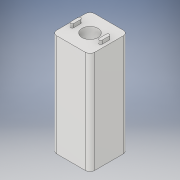
# Autodesk Inventor part: Camera Mount 30mm
Saved by Autodesk Inventor 2019 (Build 230136000, 136)
## iProperties
Created: 2020-02-21
Part Number: Camera Mount 30mm
Material: Generic
Document SubType Name: Modeling
Designer: close
Density: 1 g/cm^3
Appearance: Smooth - White
Author: close
Autodesk Inventor part; units mm, degrees
ref_plane "YZ Plane" through (0, 0, 0) normal (1, 0, 0) x (0, 1, 0)
ref_plane "XZ Plane" through (0, 0, 0) normal (0, 1, 0) x (-1, 0, 0)
ref_plane "XY Plane" through (0, 0, 0) normal (0, 0, 1) x (1, 0, 0)
sketch "Sketch1" plane through (0, 0, 0) normal (0, 1, 0) x (-1, 0, 0)
  line L0 (6, 8) -> (-6, 8)
  line L1 (-8, 6) -> (-8, -6)
  line L2 (-6, -8) -> (6, -8)
  line L3 (8, -6) -> (8, 6)
  arc A0 (8, 6) -> (6, 8) centre (6, 6) ccw
  arc A1 (-6, 8) -> (-8, 6) centre (-6, 6) ccw
  arc A2 (-8, -6) -> (-6, -8) centre (-6, -6) ccw
  arc A3 (6, -8) -> (8, -6) centre (6, -6) ccw
  point P0 (0, 0)
  point P1 (8, 8)
  point P2 (-8, 8)
  point P3 (8, -8)
  dimension "d0" = 16
  dimension "d1" = 16
  dimension "d2" = 8
  dimension "d3" = 8
  dimension "d4" = 2
  constraints: 8 end point, 8 point on circle, 8 tangent, 6 point on line, 4 centre point, 3 equal radius, 2 parallel, 1 horizontal, 1 perpendicular
  measures "d0" distance of point (8, -8) point (8, 8)
  measures "d1" distance of point (8, 8) point (-8, 8)
  measures "d2" distance from line of L0 point (0, 0)
  measures "d3" distance from line of point (0, 0) L3
  measures "d4" radius of A0
extrude "Extrusion1" add sketch "Sketch1" along normal blind 43
sketch "Sketch2" plane through (0, 0, 0) normal (0, -1, 0) x (1, 0, 0)
  line L0 (-6, 5.875) -> (-6, 3.125) construction
  line L1 (-7.375, 5.875) -> (-7.375, 3.125)
  line L2 (-4.625, 3.125) -> (-4.625, 5.875)
  arc A0 (-4.625, 5.875) -> (-7.375, 5.875) centre (-6, 5.875) ccw
  arc A1 (-7.375, 3.125) -> (-4.625, 3.125) centre (-6, 3.125) ccw
  line L3 (6, -3.125) -> (6, -5.875) construction
  line L4 (4.625, -3.125) -> (4.625, -5.875)
  line L5 (7.375, -5.875) -> (7.375, -3.125)
  arc A2 (7.375, -3.125) -> (4.625, -3.125) centre (6, -3.125) ccw
  arc A3 (4.625, -5.875) -> (7.375, -5.875) centre (6, -5.875) ccw
  point P0 (0, 0)
  point P1 (0, 0)
  point P2 (-6, 4.5)
  point P3 (6, -4.5)
  dimension "d7" = 2.75
  dimension "d8" = 12
  dimension "d9" = 6
  dimension "d10" = 9
  dimension "d11" = 4.5
  dimension "d12" = 2.75
  dimension "d13" = 2.75
  dimension "d14" = 2.75
  constraints: 16 end point, 8 point on circle, 8 tangent, 4 centre point, 3 parallel, 2 midpoint, 1 coincident, 1 vertical
  measures "d7" distance between parallel lines of L2 L1
  measures "d8" distance from line of point (6, -4.5) L0
  measures "d9" distance from line of point (0, 0) L0
  measures "d10" vertical distance of point (6, -4.5) point (-6, 4.5)
  measures "d11" vertical distance of point (0, 0) point (6, -4.5)
  measures "d12" distance of L0.start L0.end
  measures "d13" distance of L3.start L3.end
  measures "d14" distance between parallel lines of L5 L4
extrude "Extrusion2" cut sketch "Sketch2" against normal blind 2.5
hole "Hole1" at (0, 0, 0) direction (0, 1, 0) diameter 6.756 end through all clearance for "Flat Head Machine Screw (82)" size "1/4" standard "Ansi Unified Screw Threads"
sketch "Sketch3" plane through (0, 43, 0) normal (0, 1, 0) x (1, 0, 0)
  line L0 (-6, 1.5) -> (-6, -1.5) construction
  line L1 (-6.65, 1.5) -> (-6.65, -1.5)
  line L2 (-5.35, -1.5) -> (-5.35, 1.5)
  arc A0 (-5.35, 1.5) -> (-6.65, 1.5) centre (-6, 1.5) ccw
  arc A1 (-6.65, -1.5) -> (-5.35, -1.5) centre (-6, -1.5) ccw
  line L3 (6, 1.5) -> (6, -1.5) construction
  line L4 (5.35, 1.5) -> (5.35, -1.5)
  line L5 (6.65, -1.5) -> (6.65, 1.5)
  arc A2 (6.65, 1.5) -> (5.35, 1.5) centre (6, 1.5) ccw
  arc A3 (5.35, -1.5) -> (6.65, -1.5) centre (6, -1.5) ccw
  line L6 (-6, 0) -> (6, 0) construction
  line L7 (6, 8) -> (-6, 8) projected
  point P0 (0, 0)
  dimension "d25" = 0.65
  dimension "d26" = 0.65
  dimension "d27" = 3
  dimension "d29" = 0
  dimension "d30" = 12
  dimension "d31" = 6
  dimension "d32" = 3
  constraints: 18 end point, 8 point on circle, 8 tangent, 4 centre point, 4 parallel, 2 midpoint, 1 vertical
  measures "d25" radius of A0
  measures "d26" radius of A2
  measures "d27" distance of L3.start L3.end
  measures "d29" distance from line of point (0, 0) L6
  measures "d30" distance between parallel lines of L3 L0
  measures "d31" distance of L6.start point (0, 0)
  measures "d32" distance of L0.start L0.end
extrude "Extrusion3" add sketch "Sketch3" along normal blind 1.5
equation "\"d1\" = d0"
equation "\"d2\" = 0.5 * d0"
equation "\"d3\" = d2"
equation "\"d9\" = 0.5 * d8"
equation "\"d11\" = 0.5 * d10"
equation "\"d12\" = d7"
equation "\"d13\" = d7"
equation "\"d14\" = d7"
equation "\"d26\" = d25"
equation "\"d27\" = d32"
equation "\"d31\" = 0.5 * d30"
body "Solid1"
